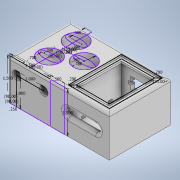
# Autodesk Inventor part: Valve Holder-3valve-withwirebox
Saved by Autodesk Inventor 2020 (Build 240168000, 168)
## iProperties
Created: 2022-01-25
Part Number: Valve Holder-3valve-withwirebox
Material: Generic
Document SubType Name: Modeling
Designer: Beaucage
Density: 1 g/cm^3
Appearance: Default
Author: Beaucage
Autodesk Inventor part; units mm, degrees
ref_plane "YZ Plane" through (0, 0, 0) normal (1, 0, 0) x (0, 1, 0)
ref_plane "XZ Plane" through (0, 0, 0) normal (0, 1, 0) x (-1, 0, 0)
ref_plane "XY Plane" through (0, 0, 0) normal (0, 0, 1) x (1, 0, 0)
sketch "Sketch1" plane through (0, 0, 0) normal (0, 1, 0) x (-1, 0, 0)
  line L0 (0, 0) -> (38.1, 0)
  line L1 (38.1, 0) -> (38.1, -38.1)
  line L2 (38.1, -38.1) -> (0, -38.1)
  line L3 (0, -38.1) -> (0, 0)
  line L4 (0, -38.1) -> (0, -31.75)
  line L5 (0, -38.1) -> (6.35, -38.1) construction
  line L6 (0, -31.75) -> (25.4, -31.75)
  line L7 (25.4, -31.75) -> (25.4, -6.35)
  line L8 (0, 0) -> (0, -38.1)
  line L9 (0, 0) -> (38.1, 0)
  line L10 (38.1, 0) -> (38.1, 12.7)
  line L11 (38.1, 12.7) -> (0, 12.7)
  line L12 (0, 12.7) -> (0, 0)
  dimension "d0" = 38.1
  dimension "d1" = 38.1
  dimension "d2" = 6.35
  dimension "d3" = 90
  dimension "d4" = 25.4
  dimension "d5" = 90
  dimension "d6" = 25.4
  dimension "d34" = 38.1
  dimension "d35" = 12.7
  constraints: 26 end point, 5 perpendicular, 4 parallel, 3 horizontal, 1 collinear
  measures "d0" distance of L1.end L2.end
  measures "d1" distance of L0.end L1.end
  measures "d2" distance of L2.end L4.end
  measures "d3" angle of L5 L4
  measures "d4" distance of L4.end L6.end
  measures "d5" angle of L4 L6
  measures "d6" distance of L6.end L7.end
  measures "d34" distance of L11.end L10.end
  measures "d35" distance of L10.end L9.end
extrude "Extrusion1" add sketch "Sketch1" along normal blind 56.896
hole "Hole1" at (-25.4, 0, -31.75) at (-25.4, 0, -6.35) direction (0, 1, 0) diameter 7.9375 depth 12.7
sketch "Sketch2" plane through (-38.1, 0, -38.1) normal (-1, 0, 0) x (0, 0, 1)
  line L0 (19.05, 0) -> (19.05, 17.78)
  line L1 (19.05, 0) -> (36.83, 0) construction
  line L2 (19.05, 17.78) -> (19.05, 27.686)
  line L3 (19.05, 17.78) -> (28.956, 17.78) construction
  line L4 (19.05, 27.686) -> (19.05, 32.766)
  line L5 (19.05, 32.766) -> (19.05, 42.672)
  circle A0 centre (19.05, 17.78) radius 9.906
  circle A1 centre (19.05, 42.672) radius 9.906
  ellipse E0 centre (19.05, 42.672) end of major axis (28.702, 42.672) minor radius 3.5267
  ellipse E1 centre (19.05, 17.78) end of major axis (28.956, 17.78) minor radius 3.6751
  line L6 (19.05, 42.672) -> (19.05, 57.404)
  line L7 (19.05, 30.226) -> (29.21, 30.226)
  line L8 (29.21, 30.226) -> (39.116, 30.226)
  circle A2 centre (39.116, 30.226) radius 9.906
  ellipse E2 centre (39.116, 30.226) end of major axis (29.21, 30.226) minor radius 3.1895
  dimension "d16" = 17.78
  dimension "d17" = 90
  dimension "d18" = 9.906
  dimension "d19" = 90
  dimension "d20" = 5.08
  dimension "d21" = 180
  dimension "d22" = 9.906
  dimension "d23" = 180
  dimension "d32" = 14.732
  dimension "d36" = 10.16
  dimension "d37" = 9.906
  dimension "d38" = 19.812
  constraints: 18 end point, 6 coincident, 5 horizontal, 3 vertical, 2 centre point, 2 collinear, 2 horizontal alignment, 2 perpendicular, 2 vertical alignment, 1 line through centre, 1 midpoint, 1 point on line, 8 other
  measures "d16" distance of L0.start L0.end
  measures "d17" angle of L1 L0
  measures "d18" distance of L0.end L2.end
  measures "d19" angle of L3 L2
  measures "d20" distance of L2.end L4.end
  measures "d21" angle of L4 L2
  measures "d22" distance of L4.end L5.end
  measures "d23" angle of L5 L4
  measures "d32" distance of L6.start L6.end
  measures "d36" distance of L7.start L7.end
  measures "d37" distance of L7.end L8.end
  measures "d38" diameter of A2
extrude "Extrusion2" cut sketch "Sketch2" against normal blind 31.75
extrude "Extrusion3" cut sketch "Sketch2" against normal blind 38.1 contours E1 L2 L0 | L0 L2 E1 | E0 L6 L5 | L5 L6 E0 | E2
sketch "Sketch3" plane through (0, 0, 0) normal (1, 0, 0) x (0, 0, -1)
  line L0 (38.1, 0) -> (38.1, 56.896) projected
  line L1 (0, 44.577) -> (38.1, 44.577)
  line L2 (38.1, 44.577) -> (38.1, 40.767)
  line L3 (38.1, 40.767) -> (0, 40.767)
  line L4 (0, 40.767) -> (0, 44.577)
  line L5 (0, 44.577) -> (38.1, 40.767) construction
  line L6 (38.1, 44.577) -> (0, 40.767) construction
  line L7 (0, 19.685) -> (38.1, 19.685)
  line L8 (38.1, 19.685) -> (38.1, 15.875)
  line L9 (38.1, 15.875) -> (0, 15.875)
  line L10 (0, 15.875) -> (0, 19.685)
  line L11 (0, 19.685) -> (38.1, 15.875) construction
  line L12 (38.1, 19.685) -> (0, 15.875) construction
  line L13 (-12.7, 0) -> (-12.7, 56.896) projected
  line L14 (0, 15.875) -> (-12.7, 15.875)
  line L15 (-12.7, 15.875) -> (-12.7, 19.685)
  line L16 (-12.7, 19.685) -> (0, 19.685)
  line L17 (0, 19.685) -> (0, 15.875)
  line L18 (0, 40.767) -> (-12.7, 40.767)
  line L19 (-12.7, 40.767) -> (-12.7, 44.577)
  line L20 (-12.7, 44.577) -> (0, 44.577)
  line L21 (0, 44.577) -> (0, 40.767)
  line L22 (-12.7, 0) -> (-12.7, 56.896) projected
  line L23 (38.1, 0) -> (38.1, 56.896) projected
  line L24 (-40.132, 28.321) -> (38.1, 28.321)
  line L25 (38.1, 28.321) -> (38.1, 32.131)
  line L26 (38.1, 32.131) -> (-40.132, 32.131)
  line L27 (-40.132, 32.131) -> (-40.132, 28.321)
  line L28 (-40.132, 28.321) -> (38.1, 32.131) construction
  line L29 (38.1, 28.321) -> (-40.132, 32.131) construction
  point P0 (0, 0)
  point P1 (19.05, 17.78)
  point P2 (19.05, 42.672)
  point P3 (-1.016, 30.226)
  point P4 (38.1, 28.321)
  dimension "d28" = 3.81
  dimension "d29" = 3.81
  dimension "d39" = 3.81
  constraints: 52 end point, 10 parallel, 6 midpoint, 5 horizontal, 5 perpendicular, 4 point on line, 2 other
  measures "d28" distance of L1.end L2.end
  measures "d29" distance of L7.end L8.end
  measures "d39" distance of L25.end L24.end
extrude "Extrusion4" cut sketch "Sketch3" against normal blind 6.35 contours L9 L10 L7 L0 | L14 L13 L16 L10 | L24 L13 L26 L0 | L24 L27 L26 L13 | L3 L4 L1 L0 | L18 L13 L20 L4
sketch "Sketch4" plane through (-38.1, 0, 12.7) normal (0, 0, 1) x (1, 0, 0)
  line L0 (38.1, 44.577) -> (38.1, 56.896) projected
  line L1 (38.1, 56.896) -> (0, 56.896)
  line L2 (0, 56.896) -> (0, 0)
  line L3 (0, 0) -> (38.1, 0)
  line L4 (38.1, 0) -> (38.1, 56.896)
  line L5 (38.1, 56.896) -> (38.1, 53.086)
  line L6 (38.1, 53.086) -> (34.29, 53.086)
  line L7 (0, 0) -> (0, 3.81)
  line L8 (0, 0) -> (0, 56.896) projected
  line L9 (0, 3.81) -> (3.81, 3.81)
  line L10 (34.29, 53.086) -> (3.81, 53.086)
  line L11 (3.81, 53.086) -> (3.81, 3.81)
  line L12 (3.81, 3.81) -> (34.29, 3.81)
  line L13 (34.29, 3.81) -> (34.29, 53.086)
  dimension "d41" = 3.81
  dimension "d42" = 3.81
  dimension "d43" = 3.81
  dimension "d44" = 3.81
  dimension "d45" = 90
  constraints: 24 end point, 4 parallel, 4 perpendicular, 2 horizontal, 2 point on line
  measures "d41" distance of L0.end L5.end
  measures "d42" distance of L5.end L6.end
  measures "d43" distance of L2.end L7.end
  measures "d44" distance of L7.end L9.end
  measures "d45" angle of L7 L9
extrude "Extrusion5" add sketch "Sketch4" along normal blind 38.1 contours L4 L3 L2 L9 L12 L13 L6 L0 | L6 L10 L11 L9 L2 L1 L0
sketch "Sketch5" plane through (-38.1, 0, 50.8) normal (0, 0, 1) x (1, 0, 0)
  line L0 (38.1, 0) -> (38.1, 56.896) projected
  line L1 (0, 0) -> (38.1, 0) projected
  line L2 (38.1, 56.896) -> (0, 56.896)
  line L3 (0, 56.896) -> (0, 0)
  line L4 (0, 0) -> (38.1, 0)
  line L5 (38.1, 0) -> (38.1, 56.896)
  constraints: 8 end point, 2 parallel, 1 horizontal, 1 perpendicular
extrude "Extrusion6" add sketch "Sketch5" along normal blind 3.81
sketch "Sketch6" plane through (0, 0, 0) normal (0, -1, 0) x (1, 0, 0)
  line L0 (0, 54.61) -> (-38.1, 54.61) projected
  line L1 (-19.05, 54.61) -> (-19.05, 29.21)
  line L2 (-19.05, 16.51) -> (-19.05, 41.91) construction
  line L3 (-15.875, 16.51) -> (-15.875, 41.91)
  line L4 (-22.225, 41.91) -> (-22.225, 16.51)
  arc A0 (-22.225, 16.51) -> (-15.875, 16.51) centre (-19.05, 16.51) ccw
  arc A1 (-15.875, 41.91) -> (-22.225, 41.91) centre (-19.05, 41.91) ccw
  point P0 (0, 0)
  dimension "d50" = 25.4
  dimension "d51" = 6.35
  constraints: 10 end point, 4 point on circle, 4 tangent, 3 midpoint, 2 centre point, 1 parallel, 1 vertical
  measures "d50" distance of L1.start L1.end
  measures "d51" diameter of A1
extrude "Extrusion7" cut sketch "Sketch6" against normal blind 3.81
sketch "Sketch7" plane through (-38.1, 0, -38.1) normal (-1, 0, 0) x (0, 0, 1)
  line L0 (50.8, 53.086) -> (88.9, 53.086) projected
  line L1 (50.8, 53.086) -> (50.8, 3.81) projected
  line L2 (88.9, 53.086) -> (50.8, 53.086)
  line L3 (50.8, 53.086) -> (50.8, 3.81)
  line L4 (50.8, 3.81) -> (88.9, 3.81)
  line L5 (88.9, 3.81) -> (88.9, 53.086)
  line L6 (88.9, 53.086) -> (85.3079, 49.4939)
  line L7 (88.9, 53.086) -> (93.98, 53.086) construction
  line L8 (50.8, 3.81) -> (54.3921, 7.4021)
  line L9 (50.8, 3.81) -> (55.88, 3.81) construction
  line L10 (85.3079, 49.4939) -> (54.3921, 49.4939)
  line L11 (54.3921, 49.4939) -> (54.3921, 7.4021)
  line L12 (54.3921, 7.4021) -> (85.3079, 7.4021)
  line L13 (85.3079, 7.4021) -> (85.3079, 49.4939)
  point P0 (38.1, 0)
  dimension "d54" = 5.08
  dimension "d55" = 135
  dimension "d56" = 5.08
  dimension "d57" = 45
  constraints: 24 end point, 4 horizontal, 4 parallel, 2 equal length, 2 perpendicular
  measures "d54" distance of L0.end L6.end
  measures "d55" angle of L6 L7
  measures "d56" distance of L1.end L8.end
  measures "d57" angle of L9 L8
extrude "Extrusion8" cut sketch "Sketch7" against normal blind 3.81 contours L13 L12 L11 L10
extrude "Extrusion9" cut sketch "Sketch7" against normal blind 1.905 contours L0 L6 L10 L11 L8 L1 | L5 L4 L8 L12 L13 L6
sketch "Sketch8" plane through (0, 56.896, 0) normal (0, 1, 0) x (1, 0, 0)
  line L0 (-38.1, -12.7) -> (-38.1, -50.8) projected
  line L1 (-38.1, -31.75) -> (-19.05, -31.75)
  line L2 (0, 38.1) -> (0, -54.61) projected
  line L3 (-24.765, -41.91) -> (-13.335, -41.91)
  line L4 (-13.335, -41.91) -> (-13.335, -21.59)
  line L5 (-13.335, -21.59) -> (-24.765, -21.59)
  line L6 (-24.765, -21.59) -> (-24.765, -41.91)
  line L7 (-24.765, -41.91) -> (-13.335, -21.59) construction
  line L8 (-13.335, -41.91) -> (-24.765, -21.59) construction
  line L9 (-20.32, -44.45) -> (-17.78, -44.45)
  line L10 (-17.78, -44.45) -> (-17.78, -19.05)
  line L11 (-17.78, -19.05) -> (-20.32, -19.05)
  line L12 (-20.32, -19.05) -> (-20.32, -44.45)
  line L13 (-20.32, -44.45) -> (-17.78, -19.05) construction
  line L14 (-17.78, -44.45) -> (-20.32, -19.05) construction
  point P0 (0, 0)
  point P1 (-20.32, -21.59)
  point P2 (-20.32, -41.91)
  point P3 (-17.78, -41.91)
  point P4 (-17.78, -21.59)
  dimension "d62" = 19.05
  dimension "d63" = 11.43
  dimension "d64" = 20.32
  dimension "d65" = 2.54
  dimension "d66" = 25.4
  constraints: 26 end point, 5 midpoint, 4 parallel, 3 perpendicular, 2 horizontal
  measures "d62" distance of L1.start L1.end
  measures "d63" distance of L5.end L4.end
  measures "d64" distance of L4.end L3.end
  measures "d65" distance of L11.end L10.end
  measures "d66" distance of L10.end L9.end
extrude "Extrusion10" cut sketch "Sketch8" against normal blind 25.4
sketch "Sketch9" plane through (0, 0, -38.1) normal (1, 0, 0) x (0, 0, -1)
  point P0 (-38.1, 0)
fillet "Fillet1" radius 3.175 16 edges at (-38.1, 28.448, -38.1) (-38.1, 56.896, 8.255) (-38.1, 0, 8.255) (-38.1, 28.448, 54.61) (-19.05, 0, 45.085) (-15.875, 0, 29.21) (-19.05, 0, 13.335) (-22.225, 0, 29.21) (-3.175, 15.875, -38.1) (-6.35, 42.672, -38.1) (-6.35, 30.226, -38.1) (-6.35, 17.78, -38.1) (-3.175, 28.321, -38.1) (-3.175, 32.131, -38.1) (-3.175, 40.767, -38.1) (-3.175, 44.577, -38.1)
body "Solid1"
